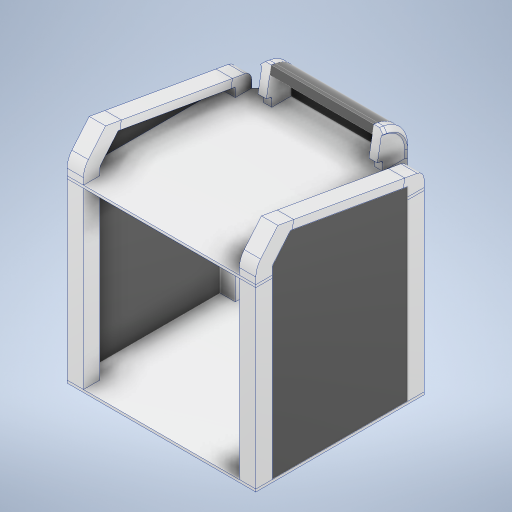
# Autodesk Inventor part: RevII Refined Printer Envelope Study
Saved by Autodesk Inventor 2024 (Build 280153000, 153)
## iProperties
Created: 2024-07-22
Part Number: RevII Refined Printer Envelope Study
Material: Generic
Document SubType Name: Modeling
Designer: Ishaan
Density: 1 g/cm^3
Appearance: Smooth - Black
Author: Ishaan
Autodesk Inventor part; units mm, degrees
ref_plane "YZ Plane" through (0, 0, 0) normal (1, 0, 0) x (0, 1, 0)
ref_plane "XZ Plane" through (0, 0, 0) normal (0, 1, 0) x (-1, 0, 0)
ref_plane "XY Plane" through (0, 0, 0) normal (0, 0, 1) x (1, 0, 0)
sketch "Sketch1" plane through (0, 0, 0) normal (0, 0, 1) x (1, 0, 0)
  line L0 (230, -205) -> (-230, -205)
  line L1 (-230, -205) -> (-230, 205)
  line L2 (-230, 205) -> (230, 205)
  line L3 (230, 205) -> (230, -205)
  line L4 (230, -205) -> (-230, 205) construction
  line L5 (-230, -205) -> (230, 205) construction
  line L6 (-190, 205) -> (-139.1421, 255.8579)
  line L7 (-139.1421, 255.8579) -> (139.1421, 255.8579)
  line L8 (139.1421, 255.8579) -> (190, 205)
  line L9 (139.1421, 255.8579) -> (135.0218, 245.9106) construction
  line L10 (135, 255.8579) -> (135, 245.8579) construction
  line L11 (230, 205) -> (190, 205)
  line L12 (190, 205) -> (190, 165)
  line L13 (190, 165) -> (230, 165)
  line L14 (230, 165) -> (230, 205)
  line L15 (-150, 105) -> (150, 105)
  line L16 (150, 105) -> (150, -145)
  line L17 (150, -145) -> (-150, -145)
  line L18 (-150, -145) -> (-150, 105)
  line L19 (-230, -205) -> (-190, -205)
  line L20 (-190, -205) -> (-190, -165)
  line L21 (-190, -165) -> (-230, -165)
  line L22 (-230, -165) -> (-230, -205)
  line L23 (230, -205) -> (190, -205)
  line L24 (190, -205) -> (190, -165)
  line L25 (190, -165) -> (230, -165)
  line L26 (230, -165) -> (230, -205)
  line L27 (-230, 205) -> (-190, 205)
  line L28 (-190, 205) -> (-190, 165)
  line L29 (-190, 165) -> (-230, 165)
  line L30 (-230, 165) -> (-230, 205)
  line L31 (-40, 205) -> (40, 205)
  line L32 (40, 205) -> (40, 165)
  line L33 (40, 165) -> (-40, 165)
  line L34 (-40, 165) -> (-40, 205)
  line L35 (125, 255.8579) -> (135, 255.8579)
  line L36 (135, 255.8579) -> (135, 235.8579)
  line L37 (135, 235.8579) -> (125, 235.8579)
  line L38 (125, 235.8579) -> (125, 255.8579)
  line L39 (149.1421, 245.8579) -> (142.0711, 252.9289)
  line L40 (142.0711, 252.9289) -> (127.9289, 238.7868)
  line L41 (127.9289, 238.7868) -> (135, 231.7157)
  line L42 (135, 231.7157) -> (149.1421, 245.8579)
  line L43 (135, 205) -> (132, 205)
  line L44 (132, 205) -> (132, 231)
  line L45 (132, 231) -> (135, 231)
  line L46 (135, 231) -> (135, 205)
  line L47 (135, 205) -> (95, 205)
  line L48 (95, 205) -> (95, 185)
  line L49 (95, 185) -> (135, 185)
  line L50 (135, 185) -> (135, 205)
  line L51 (-222, 75) -> (-132, 75)
  line L52 (-132, 75) -> (-132, -145)
  line L53 (-132, -145) -> (-222, -145)
  line L54 (-222, -145) -> (-222, 75)
  line L55 (-135, 205) -> (-95, 205)
  line L56 (-95, 205) -> (-95, 185)
  line L57 (-95, 185) -> (-135, 185)
  line L58 (-135, 185) -> (-135, 205)
  line L59 (-149.1421, 245.8579) -> (-142.0711, 252.9289)
  line L60 (-142.0711, 252.9289) -> (-127.9289, 238.7868)
  line L61 (-127.9289, 238.7868) -> (-135, 231.7157)
  line L62 (-135, 231.7157) -> (-149.1421, 245.8579)
  line L63 (-125, 255.8579) -> (-135, 255.8579)
  line L64 (-135, 255.8579) -> (-135, 235.8579)
  line L65 (-135, 235.8579) -> (-125, 235.8579)
  line L66 (-125, 235.8579) -> (-125, 255.8579)
  point P0 (0, 0)
  point P1 (0, 105)
  point P2 (0, 205)
  point P3 (-135, 245.8579)
  point P4 (130.8579, 235.8579)
  point P5 (-130.8579, 235.8579)
  point P6 (40, 205)
  dimension "d0" = 460
  dimension "d1" = 410
  dimension "d2" = 40
  dimension "d3" = 40
  dimension "d4" = 135
  dimension "d5" = 135
  dimension "d30" = 67.5
  dimension "d32" = 10
  dimension "d34" = 50.8579
  dimension "d35" = 40
  dimension "d36" = 40
  dimension "d37" = 300
  dimension "d38" = 250
  dimension "d39" = 60
  dimension "d40" = 40
  dimension "d41" = 40
  dimension "d42" = 40
  dimension "d43" = 40
  dimension "d44" = 40
  dimension "d45" = 40
  dimension "d46" = 80
  dimension "d47" = 40
  dimension "d48" = 10
  dimension "d50" = 10
  dimension "d51" = 3
  dimension "d52" = 26
  dimension "d53" = 40
  dimension "d54" = 20
  dimension "d55" = 55
  dimension "d56" = 105
  dimension "d57" = 90
  dimension "d58" = 220
  dimension "d59" = 8
  dimension "d60" = 20
  dimension "d61" = 55
  dimension "d65" = 55
  constraints: 134 end point, 30 parallel, 15 perpendicular, 13 horizontal, 12 point on line, 9 midpoint, 6 equal length, 1 collinear, 1 vertical, 1 vertical alignment
  measures "d0" distance of L1.end L2.end
  measures "d1" distance of L0.end L1.end
  measures "d2" distance from line of L3 L8.end
  measures "d3" distance from line of L6.start L1
  measures "d4" angle of L7 L6
  measures "d5" angle of L8 L7
  measures "d30" angle of L9 L7
  measures "d32" distance of L10.end L10.start
  measures "d34" distance between parallel lines of L2 L7
  measures "d35" distance of L13.end L12.end
  measures "d36" distance of L12.end L11.end
  measures "d37" distance of L16.end L17.end
  measures "d38" distance of L15.end L16.end
  measures "d39" distance between parallel lines of L0 L17
  measures "d40" distance of L21.end L20.end
  measures "d41" distance of L20.end L19.end
  measures "d42" distance of L24.end L25.end
  measures "d43" distance of L23.end L24.end
  measures "d44" distance of L28.end L29.end
  measures "d45" distance of L27.end L28.end
  measures "d46" distance of L32.end L33.end
  measures "d47" distance of L31.end L32.end
  measures "d48" distance of L36.end L37.end
  measures "d50" distance of L40.end L41.end
  measures "d51" distance of L44.end L45.end
  measures "d52" distance of L45.end L43.start
  measures "d53" distance of L49.end L48.end
  measures "d54" distance of L48.end L47.end
  measures "d55" distance between parallel lines of L48 L32
  measures "d56" distance between parallel lines of L3 L38
  measures "d57" distance of L52.end L53.end
  measures "d58" distance of L51.end L52.end
  measures "d59" distance between parallel lines of L1 L54
  measures "d60" distance between parallel lines of L21 L53
  measures "d61" distance between parallel lines of L12 L50
  measures "d65" distance between parallel lines of L34 L56
extrude "Extrusion1" add sketch "Sketch1" along normal blind 450 contours L0 L24 L25 L3 | L0 L20 L21 L1 L29 L28 L2 L58 L57 L56 L34 L33 L32 L48 L49 L50 L12 L13 L3 L25 L24 | L0 L1 L21 L20 | L13 L12 L2 L3 | L2 L46 L45 L44 L6 L62 L61 L65 L66 L7 L38 L37 L41 L42 L8 | L1 L2 L28 L29 | L50 L49 L48 L2 | L2 L44 L45 L46 | L42 L41 L37 L36 L40 L8 | L40 L36 L7 L8 | L40 L41 L37 L38 L7 L36 | L36 L37 L41 L40 | L2 L56 L57 L58 | L6 L60 L64 L65 L61 L62 | L32 L33 L34 L2 | L6 L7 L64 L60 | L64 L7 L66 L65 L61 L60 | L60 L61 L65 L64 | L15 L16 L17 L52 L51 L18 | L51 L52 L17 L18 | L18 L53 L54 L51
sketch "Sketch2" plane through (0, 0, 450) normal (0, 0, 1) x (1, 0, 0)
  line L0 (-139.1421, 255.8579) -> (-190, 205) projected
  line L1 (-190, 205) -> (-230, 205) projected
  line L2 (-230, 205) -> (-230, -205) projected
  line L3 (-230, -205) -> (230, -205) projected
  line L4 (230, -205) -> (230, 205) projected
  line L5 (230, 205) -> (190, 205) projected
  line L6 (190, 205) -> (139.1421, 255.8579) projected
  line L7 (139.1421, 255.8579) -> (-139.1421, 255.8579) projected
  line L8 (230, 185) -> (-230, 185)
  point P0 (0, 0)
  dimension "d9" = 20
  constraints: 2 end point, 2 point on line
  measures "d9" distance between parallel lines of L8 L1
revolve "Revolution1" add sketch "Sketch2" angle 80 about axis through (230, 185, 450) along (1, 0, 0) contours L7 L6 L5 L4 L8 L2 L1 L0
sketch "Sketch3" plane through (-230, 185, 450) normal (0, -0.9848078, 0.1736482) x (1, 0, 0)
  line L0 (0, 20) -> (0, 0) projected
  line L1 (460, 0) -> (0, 0) projected
  line L2 (460, 0) -> (460, 20) projected
  line L3 (460, 20) -> (420, 20) projected
  line L4 (420, 20) -> (369.1421, 70.8579) projected
  line L5 (369.1421, 70.8579) -> (90.8579, 70.8579) projected
  line L6 (90.8579, 70.8579) -> (40, 20) projected
  line L7 (40, 20) -> (0, 20) projected
  point P0 (230, -475.2884)
ref_plane "Work Plane4" through (-230, -212.6604, 456.4279) normal (0, 0.7660444, -0.6427876) x (1, 0, 0)
ref_plane "Work Plane3" through (-230, -205, 450) normal (0, 0.7660444, -0.6427876) x (1, 0, 0)
extrude "Extrusion5" add sketch "Sketch3" along normal up to surface surface through (-230, -212.6604, 456.4279) normal (0, 0.7660444, -0.6427876)
sketch "Sketch6" plane through (-230, -205, 0) normal (-1, 0, 0) x (0, 0, 1)
  line L0 (0, 410) -> (0, 0) projected
  line L1 (0, 0) -> (450, 0) projected
  line L2 (450, 390) -> (450, 0) projected
  line L3 (450, 390) -> (511.9094, 38.8941) projected
  line L4 (529.6005, 53.7387) -> (511.9094, 38.8941) projected
  line L5 (469.6962, 393.473) -> (529.6005, 53.7387) projected
  arc A0 (469.6962, 393.473) -> (450, 410) centre (450, 390) ccw projected
  line L6 (0, 410) -> (450, 410) projected
  line L7 (511.9094, 38.8941) -> (465.5572, 0)
  line L8 (465.5572, 0) -> (450, 0)
  point P0 (0, 205)
  constraints: 4 end point, 1 collinear, 1 horizontal
extrude "Extrusion6" add sketch "Sketch6" against normal up to surface (460 mm away) contours L2 L3 L7 L8
fillet "Fillet1" radius 50 1 edges at (0, -205, 465.5572)
fillet "Fillet3" radius 2 6 edges at (-190, 200.3209, 462.8558) (-190, 205, 225) (-190, 18.6058, 499.6483) (190, 200.3209, 462.8558) (190, 205, 225) (190, 18.6058, 499.6483)
fillet "Fillet4" radius 2 13 edges at (0, -113.5133, 574.5869) (-139.1421, 239.2803, 495.5466) (-139.1421, 255.8579, 225) (-139.1421, 41.8955, 547.1841) (-190.0631, -151.1483, 529.7351) (-210.4142, -151.2613, 529.6005) (-164.2782, -132.1699, 552.3528) (190.0631, -151.1483, 529.7351) (210.4142, -151.2613, 529.6005) (164.2782, -132.1699, 552.3528) (139.1421, 239.2803, 495.5466) (139.1421, 255.8579, 225) (139.1421, 41.8955, 547.1841)
fillet "Fillet5" radius 2 14 edges at (-230, -151.1555, 529.3097) (-230, 19.1744, 499.5481) (-230, 200.3209, 462.8558) (-230, 205, 225) (-230, -201.9846, 464.4597) (-230, -205, 223.6794) (-230, -172.6529, 504.107) (230, -151.1555, 529.3097) (230, 19.1744, 499.5481) (230, 200.3209, 462.8558) (230, 205, 225) (230, -201.9846, 464.4597) (230, -205, 223.6794) (230, -172.6529, 504.107)
extrude "Extrusion7" add sketch "Sketch1" against normal blind 6.35 separate body contours L0 L24 L25 L3 | L0 L20 L21 L1 L29 L28 L2 L58 L57 L56 L34 L33 L32 L48 L49 L50 L12 L13 L3 L25 L24 | L0 L1 L21 L20 | L13 L12 L2 L3 | L2 L46 L45 L44 L6 L62 L61 L65 L66 L7 L38 L37 L41 L42 L8 | L1 L2 L28 L29 | L50 L49 L48 L2 | L2 L44 L45 L46 | L42 L41 L37 L36 L40 L8 | L40 L36 L7 L8 | L40 L41 L37 L38 L7 L36 | L36 L37 L41 L40 | L2 L56 L57 L58 | L6 L60 L64 L65 L61 L62 | L32 L33 L34 L2 | L6 L7 L64 L60 | L64 L7 L66 L65 L61 L60 | L60 L61 L65 L64 | L15 L16 L17 L52 L51 L18 | L51 L52 L17 L18 | L18 L53 L54 L51
sketch "Sketch8" plane through (0, 0, -6.35) normal (0, 0, -1) x (1, 0, 0)
  line L0 (230, -205) -> (230, 205) projected
  line L1 (-230, -205) -> (-190, -205) projected
  line L2 (139.1421, -255.8579) -> (190, -205) projected
  line L3 (-139.1421, -255.8579) -> (139.1421, -255.8579) projected
  line L4 (-190, -205) -> (-139.1421, -255.8579) projected
  line L5 (190, -205) -> (230, -205) projected
  line L6 (-230, 205) -> (-230, -205) projected
  line L7 (230, 205) -> (-230, 205) projected
  point P0 (0, 0)
extrude "Extrusion8" add sketch "Sketch1" along normal blind 425 separate body contours L0 L24 L25 L3 | L0 L1 L21 L20 | L13 L12 L2 L3 | L1 L2 L28 L29 | L50 L49 L48 L2 | L42 L41 L37 L36 L40 L8 | L40 L36 L7 L8 | L40 L41 L37 L38 L7 L36 | L36 L37 L41 L40 | L2 L56 L57 L58 | L6 L60 L64 L65 L61 L62 | L32 L33 L34 L2 | L6 L7 L64 L60 | L64 L7 L66 L65 L61 L60 | L60 L61 L65 L64
sketch "Sketch9" plane through (0, 0, 425) normal (0, 0, 1) x (1, 0, 0)
  line L0 (230, -205) -> (230, 205) projected
  line L1 (230, 205) -> (190, 205) projected
  line L2 (190, 205) -> (139.1421, 255.8579) projected
  line L3 (139.1421, 255.8579) -> (-139.1421, 255.8579) projected
  line L4 (-139.1421, 255.8579) -> (-190, 205) projected
  line L5 (-190, 205) -> (-230, 205) projected
  line L6 (-230, 205) -> (-230, -205) projected
  line L7 (-230, -205) -> (230, -205) projected
  point P0 (0, 0)
extrude "Extrusion9" add sketch "Sketch9" along normal blind 6.35 separate body
sketch "Sketch10" plane through (-230, -205, 425) normal (-1, 0, 0) x (0, 0, 1)
  line L0 (25, 410) -> (-425, 410) projected
  line L1 (-425, 410) -> (25, 410) projected
  arc A0 (44.6962, 393.473) -> (25, 410) centre (25, 390) ccw projected
  arc A1 (44.6962, 393.473) -> (25, 410) centre (25, 390) ccw projected
  line L2 (104.4, 54.8758) -> (44.6962, 393.473) projected
  line L3 (44.6962, 393.473) -> (104.4, 54.8758) projected
  line L4 (103.7159, 52.9964) -> (54.4981, 11.6978) projected
  line L5 (104.7522, 53.866) -> (103.7159, 52.9964) projected
  line L6 (148.7023, 90.7445) -> (104.7522, 53.866) projected
  line L7 (104.7522, 53.866) -> (148.7023, 90.7445) projected
  line L8 (103.7159, 52.9964) -> (104.7522, 53.866) projected
  line L9 (54.4981, 11.6978) -> (103.7159, 52.9964) projected
  arc A2 (22.3587, 0) -> (54.4981, 11.6978) centre (22.3587, 50) ccw projected
  arc A3 (22.3587, 0) -> (54.4981, 11.6978) centre (22.3587, 50) ccw projected
  line L10 (22.3587, 0) -> (-425, 0) projected
  line L11 (-425, 0) -> (22.3587, 0) projected
  line L12 (6.35, 410) -> (6.35, 0) projected
  line L13 (6.35, 370) -> (26.8483, 370)
  line L14 (50.0591, 363.0584) -> (30.3629, 359.5855)
  line L15 (30.3629, 359.5855) -> (28.818, 368.3473)
  arc A4 (28.818, 368.3473) -> (26.8483, 370) centre (26.8483, 368) ccw
  line L16 (6.35, 40) -> (22.3587, 40)
  line L17 (28.7866, 42.3396) -> (78.0044, 83.6382)
  line L18 (78.6885, 85.5176) -> (78.1162, 88.7633)
  line L19 (78.1162, 88.7633) -> (97.8123, 92.2363)
  line L20 (104.4, 54.8758) -> (104.6005, 53.7387)
  arc A5 (22.3587, 40) -> (28.7866, 42.3396) centre (22.3587, 50) ccw
  arc A6 (78.0044, 83.6382) -> (78.6885, 85.5176) centre (76.7188, 85.1703) ccw
  line L21 (30.3629, 359.5855) -> (78.1162, 88.7633) construction
  line L22 (54.2395, 224.1744) -> (74.5481, 224.1744) construction
  line L23 (30.3629, 359.5855) -> (78.1162, 88.7633)
  point P0 (-425, 205)
  point P1 (104.6005, 53.7387)
  point P2 (104.4, 54.8758)
  point P3 (97.8123, 92.2363)
  dimension "d70" = 20
  dimension "d71" = 40
  dimension "d72" = 20
  dimension "d73" = 2
  dimension "d74" = 40
  dimension "d76" = 2
  dimension "d77" = 275
  constraints: 22 end point, 6 point on circle, 6 tangent, 5 point on line, 3 centre point, 3 collinear, 3 horizontal, 2 midpoint, 2 parallel, 2 perpendicular, 1 concentric
  measures "d70" distance of L14.start L14.end
  measures "d71" distance between parallel lines of L13 L0
  measures "d72" radius of A0
  measures "d73" radius of A4
  measures "d74" distance between parallel lines of L10 L16
  measures "d76" radius of A6
  measures "d77" distance between parallel lines of L19 L14
extrude "Extrusion10" add sketch "Sketch10" against normal blind 40 separate body contours A0 L2 L14 L15 A4 L13 L12 L0 | L16 A5 L17 A6 L18 L19 L2 L20 L5 L4 A2 L10 L12
mirror "Mirror1" about plane through (0, 0, 0) normal (1, 0, 0) of "Extrusion10" bodies 5
extrude "Extrusion11" add sketch "Sketch10" against normal blind 40 separate body contours L2 L19 L23 L14
mirror "Mirror2" about plane through (0, 0, 0) normal (1, 0, 0) of "Extrusion11" bodies 6
sketch "Sketch12" plane through (-230, -205, 425) normal (-1, 0, 0) x (0, 0, 1)
  line L0 (0, 410) -> (0, 0) projected
  line L1 (0, 0) -> (6.35, 0) projected
  line L2 (6.35, 410) -> (6.35, 0) projected
  line L3 (0, 410) -> (6.35, 410) projected
  line L4 (28.818, 368.3473) -> (30.3629, 359.5855) projected
  line L5 (30.3629, 359.5855) -> (50.0591, 363.0584) projected
  line L6 (50.0591, 363.0584) -> (44.6962, 393.473) projected
  arc A0 (44.6962, 393.473) -> (25, 410) centre (25, 390) ccw projected
  line L7 (25, 410) -> (6.35, 410) projected
  line L8 (6.35, 410) -> (6.35, 370) projected
  line L9 (6.35, 370) -> (26.8483, 370) projected
  arc A1 (28.818, 368.3473) -> (26.8483, 370) centre (26.8483, 368) ccw projected
  line L10 (-425, 40) -> (-425, 0) projected
  line L11 (-425, 0) -> (0, 0) projected
  line L12 (0, 40) -> (0, 0) projected
  line L13 (-425, 40) -> (0, 40) projected
  line L14 (0, 40) -> (6.35, 40)
  line L15 (6.35, 40) -> (6.35, 370)
  line L16 (6.35, 370) -> (0, 370)
  line L17 (0, 370) -> (0, 40)
  point P0 (-425, 205)
  constraints: 8 end point, 2 parallel, 1 horizontal, 1 perpendicular
extrude "Extrusion12" cut sketch "Sketch12" against normal blind 3.5 contours L16 L2 L14 L0 bodies 4
mirror "Mirror3" about plane through (0, 0, 0) normal (1, 0, 0) of "Extrusion12" bodies 4
sketch "Sketch13" plane through (230, -205, 431.35) normal (1, 0, 0) x (0, 0, -1)
  line L0 (431.35, 40) -> (6.35, 40) projected
  line L1 (6.35, 40) -> (0, 40) projected
  line L2 (-16.0087, 40) -> (0, 40) projected
  arc A0 (-22.4366, 42.3396) -> (-16.0087, 40) centre (-16.0087, 50) ccw projected
  line L3 (-71.6544, 83.6382) -> (-22.4366, 42.3396) projected
  arc A1 (-72.3385, 85.5176) -> (-71.6544, 83.6382) centre (-70.3688, 85.1703) ccw projected
  line L4 (-71.7662, 88.7633) -> (-72.3385, 85.5176) projected
  line L5 (-24.0129, 359.5855) -> (-71.7662, 88.7633) projected
  line L6 (-22.468, 368.3473) -> (-24.0129, 359.5855) projected
  arc A2 (-20.4983, 370) -> (-22.468, 368.3473) centre (-20.4983, 368) ccw projected
  line L7 (0, 370) -> (-20.4983, 370) projected
  line L8 (0, 370) -> (6.35, 370) projected
  line L9 (431.35, 370) -> (6.35, 370) projected
  line L10 (431.35, 40) -> (431.35, 370)
  line L11 (437.7, 410) -> (437.7, 0) projected
  line L12 (6.35, 369.5) -> (0, 369.5)
  line L13 (0, 369.5) -> (-20.4983, 369.5)
  arc A3 (-20.4983, 369.5) -> (-21.9756, 368.2605) centre (-20.4983, 368) ccw
  line L14 (-21.9756, 368.2605) -> (-23.5205, 359.4986)
  line L15 (-23.5205, 359.4986) -> (-71.2737, 88.6765)
  line L16 (-71.2737, 88.6765) -> (-71.8461, 85.4308)
  arc A4 (-71.8461, 85.4308) -> (-71.333, 84.0212) centre (-70.3688, 85.1703) ccw
  line L17 (-71.333, 84.0212) -> (-22.1152, 42.7226)
  arc A5 (-22.1152, 42.7226) -> (-16.0087, 40.5) centre (-16.0087, 50) ccw
  line L18 (-16.0087, 40.5) -> (0, 40.5)
  line L19 (0, 40.5) -> (6.35, 40.5)
  line L20 (6.35, 40.5) -> (430.85, 40.5)
  line L21 (430.85, 40.5) -> (430.85, 369.5)
  line L22 (430.85, 369.5) -> (6.35, 369.5)
  point P0 (431.35, 205)
  dimension "d84" = 0.5
  constraints: 24 end point, 6 point on circle, 3 centre point, 1 parallel, 13 other
  measures "d84" distance between parallel lines of L9 L22
extrude "Extrusion13" add sketch "Sketch13" against normal blind 3.175 separate body contours L22 L21 L20 L19 L18 A5 L17 A4 L16 L15 L14 A3 L13 L12
mirror "Mirror4" about plane through (0, 0, 0) normal (1, 0, 0) of "Extrusion13" bodies 7
sketch "Sketch14" plane through (0, 0, 0) normal (1, 0, 0) x (0, 1, 0)
  line L0 (-205, 0) -> (-205, 447.3587) projected
  arc A0 (-193.3022, 479.4981) -> (-205, 447.3587) centre (-155, 447.3587) ccw projected
  line L1 (-193.3022, 479.4981) -> (-114.2555, 573.7023) projected
  arc A1 (-112.3761, 574.3864) -> (-114.2555, 573.7023) centre (-112.7234, 572.4168) ccw projected
  line L2 (-112.3761, 574.3864) -> (197.3043, 519.7814) projected
  arc A2 (255.8579, 450) -> (197.3043, 519.7814) centre (185, 450) ccw projected
  line L3 (255.8579, 450) -> (255.8579, 0) projected
  line L4 (255.8579, 0) -> (-205, 0) projected
  line L5 (-205, -6.35) -> (-205, 0) projected
  line L6 (-205, 0) -> (255.8579, 0) projected
  line L7 (255.8579, 0) -> (255.8579, -6.35) projected
  line L8 (255.8579, -6.35) -> (-205, -6.35) projected
  line L9 (205, 425) -> (205, 0) projected
  line L10 (205, 0) -> (165, 0) projected
  line L11 (165, 0) -> (165, 425) projected
  line L12 (165, 425) -> (205, 425) projected
  line L13 (-205, 431.35) -> (255.8579, 431.35) projected
  line L14 (255.8579, 431.35) -> (255.8579, 425) projected
  line L15 (255.8579, 425) -> (-205, 425) projected
  line L16 (-205, 425) -> (-205, 431.35) projected
  line L17 (187.4563, 521.5179) -> (183.9833, 501.8217)
  line L18 (235.8579, 431.35) -> (235.8579, 450)
  line L19 (183.9833, 501.8217) -> (193.8314, 500.0852)
  arc A3 (235.8579, 450) -> (193.8314, 500.0852) centre (185, 450) ccw
  point P0 (0, 0)
  dimension "d88" = 10
  dimension "d89" = 20
  constraints: 6 end point, 2 perpendicular, 2 point on circle, 2 point on line, 2 tangent, 1 centre point, 1 concentric, 1 vertical
  measures "d88" distance from line of L2.end L17
  measures "d89" distance of L17.start L17.end
extrude "Extrusion14" add sketch "Sketch14" along normal up to surface (125 mm away) separate body contours L18 A3 L19 L17 L2 A2 L3 L13
extrude "Extrusion15" add sketch "Sketch14" against normal up to surface (125 mm away) contours L18 A3 L19 L17 L2 A2 L3 L13 bodies 8
sketch "Sketch15" plane through (-139.1421, 255.8579, 425) normal (0, 1, 0) x (1, 0, 0)
  line L0 (278.2843, 0) -> (0, 0) projected
  line L1 (0, 0) -> (0, -6.35) projected
  line L2 (278.2843, -6.35) -> (0, -6.35) projected
  line L3 (278.2843, 0) -> (278.2843, -6.35) projected
  line L4 (278.2843, 425) -> (264.1421, 425) projected
  line L5 (264.1421, 425) -> (264.1421, 0) projected
  line L6 (278.2843, 0) -> (264.1421, 0) projected
  line L7 (278.2843, 425) -> (278.2843, 0) projected
  line L8 (14.1421, 425) -> (0, 425) projected
  line L9 (0, 425) -> (0, 0) projected
  line L10 (14.1421, 0) -> (0, 0) projected
  line L11 (14.1421, 425) -> (14.1421, 0) projected
  line L12 (14.1421, 0) -> (264.1421, 0)
  line L13 (264.1421, 0) -> (264.1421, -6.35)
  line L14 (264.1421, -6.35) -> (14.1421, -6.35)
  line L15 (14.1421, -6.35) -> (14.1421, 0)
  point P0 (139.1421, 425)
  constraints: 8 end point, 2 parallel, 2 point on line, 1 horizontal, 1 perpendicular
extrude "Extrusion16" cut sketch "Sketch15" against normal blind 3.5 contours L13 L2 L15 L0 bodies 4
sketch "Sketch16" plane through (125, 255.8579, 0) normal (0, 1, 0) x (1, 0, 0)
  line L0 (0, -425) -> (0, -431.35) projected
  line L1 (14.1421, -431.35) -> (0, -431.35) projected
  line L2 (14.1421, -425) -> (14.1421, -431.35) projected
  line L3 (14.1421, -425) -> (0, -425) projected
  line L4 (-250, 0) -> (-264.1421, 0) projected
  line L5 (-264.1421, 0) -> (-264.1421, -425) projected
  line L6 (-250, -425) -> (-264.1421, -425) projected
  line L7 (-250, 0) -> (-250, -425) projected
  line L8 (-250, -431.35) -> (0, -431.35) projected
  line L9 (0, -431.35) -> (-250, -431.35)
  line L10 (-250, -431.35) -> (-250, 0)
  line L11 (-250, 0) -> (0, 0)
  line L12 (0, 0) -> (0, -431.35)
  line L13 (-0.5, -0.5) -> (-249.5, -0.5)
  line L14 (-249.5, -0.5) -> (-249.5, -430.85)
  line L15 (-249.5, -430.85) -> (-0.5, -430.85)
  line L16 (-0.5, -430.85) -> (-0.5, -0.5)
  point P0 (-125, 0)
  dimension "d96" = 0.5
  constraints: 16 end point, 4 parallel, 2 perpendicular, 1 horizontal, 3 other
  measures "d96" distance between parallel lines of L11 L13
extrude "Extrusion17" add sketch "Sketch16" against normal blind 3.175 separate body contours L16 L15 L14 L13
sketch "Sketch17" plane through (0, 0, 431.35) normal (0, 0, 1) x (1, 0, 0)
  line L0 (135, 231.7157) -> (149.1421, 245.8579) projected
  line L1 (135, 231.7157) -> (149.1421, 245.8579) projected
  line L2 (145.6066, 242.3223) -> (145.6066, 188.9073)
  line L3 (125, 183.9833) -> (125, 193.8314) projected
  line L4 (145.6066, 188.9073) -> (125, 188.9073)
  line L5 (125, 235.8579) -> (125, 255.8579) projected
  line L6 (125, 255.8579) -> (125, 188.9073)
  line L7 (125, 255.8579) -> (125, 252.3579) projected
  line L8 (125, 252.3579) -> (-125, 252.3579) projected
  line L9 (-125, 252.3579) -> (-125, 255.8579) projected
  line L10 (-125, 255.8579) -> (-139.1421, 255.8579) projected
  line L11 (-139.1421, 255.8579) -> (-190, 205) projected
  line L12 (-190, 205) -> (-230, 205) projected
  line L13 (-230, 205) -> (-230, 165) projected
  line L14 (-230, 165) -> (-226.5, 165) projected
  line L15 (-226.5, 165) -> (-226.5, -165) projected
  line L16 (-226.5, -165) -> (-230, -165) projected
  line L17 (-230, -165) -> (-230, -205) projected
  line L18 (-230, -205) -> (230, -205) projected
  line L19 (230, -205) -> (230, -165) projected
  line L20 (230, -165) -> (226.5, -165) projected
  line L21 (226.5, -165) -> (226.5, 165) projected
  line L22 (226.5, 165) -> (230, 165) projected
  line L23 (230, 165) -> (230, 205) projected
  line L24 (230, 205) -> (190, 205) projected
  line L25 (190, 205) -> (139.1421, 255.8579) projected
  line L26 (139.1421, 255.8579) -> (125, 255.8579) projected
  point P0 (0, 0)
  dimension "d99" = 5
  constraints: 6 end point, 1 collinear, 1 midpoint, 1 parallel, 1 perpendicular, 1 point on line
  measures "d99" distance of L0.end L2.start
extrude "Extrusion18" add sketch "Sketch17" along normal blind 18.65 separate body contours L2 L4 L3 L6 L5 L26 L25 L0
sketch "Sketch18" plane through (0, 0, 450) normal (0, 0, 1) x (1, 0, 0)
  line L0 (125, 255.8579) -> (125, 188.9073) projected
  line L1 (125, 188.9073) -> (145.6066, 188.9073) projected
  line L2 (145.6066, 188.9073) -> (145.6066, 242.3223) projected
  line L3 (145.6066, 242.3223) -> (149.1421, 245.8579) projected
  line L4 (149.1421, 245.8579) -> (139.1421, 255.8579) projected
  line L5 (139.1421, 255.8579) -> (125, 255.8579) projected
  point P0 (0, 0)
revolve "Revolution2" add sketch "Sketch18" angle 80 about axis through (230, 185, 450) along (1, 0, 0) bodies 10
sketch "Sketch19" plane through (125, 185.6785, 453.848) normal (0, -0.9848078, 0.1736482) x (1, 0, 0)
  line L0 (0, 0) -> (20.6066, 0) projected
  line L1 (20.6066, 0) -> (20.6066, 53.415) projected
  line L2 (20.6066, 53.415) -> (24.1421, 56.9505) projected
  line L3 (24.1421, 56.9505) -> (14.1421, 66.9505) projected
  line L4 (14.1421, 66.9505) -> (0, 66.9505) projected
  line L5 (0, 66.9505) -> (0, 0) projected
  point P0 (-125, -479.1957)
extrude "Extrusion19" add sketch "Sketch19" along normal up to surface (10 mm away) bodies 10
mirror "Mirror5" about plane through (0, 0, 0) normal (1, 0, 0) bodies 10
equation "\"d30\" = 0.5 * d5"
body "Solid1"
